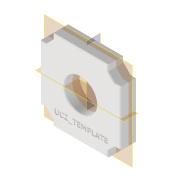
# Autodesk Inventor part: 20_Cube_Insert_Filter_25mm
Saved by Autodesk Inventor 2022 (Build 260153000, 153)
## iProperties
Created: 2019-07-01
Part Number: 20_Cube_Insert_Filter_25mm
Material: Generic
Document SubType Name: Modeling
Designer: diederichbenedict
Density: 1 g/cm^3
Appearance: Default
Author: diederichbenedict
Autodesk Inventor part; units mm, degrees
ref_plane "YZ Plane" through (0, 0, 0) normal (1, 0, 0) x (0, 1, 0)
ref_plane "XZ Plane" through (0, 0, 0) normal (0, 1, 0) x (-1, 0, 0)
ref_plane "Work Plane1" through (-56.3599, 0, 22) normal (0, 0, -1) x (-1, 0, 0)
sketch "Sketch1" plane through (-56.3599, 0, 22) normal (0, 0, -1) x (-1, 0, 0)
  line L0 (-4.0299, -0.3538) -> (-2.2322, 1.4439) construction
  arc A0 (-1.4439, 2.2322) -> (-2.2322, 1.4439) centre (-0.9299, 0.9299) ccw construction
  line L1 (-1.4439, 2.2322) -> (0.3538, 4.0299) construction
  line L2 (-37.8299, 42.8299) -> (-37.8299, 37.8299) construction
  line L3 (-37.8299, 37.8299) -> (-42.9208, 37.8299) construction
  line L4 (-37.8299, 42.2137) -> (-37.8299, 45.8299) construction
  line L5 (-37.8299, 45.8299) -> (-4.0299, 45.8299) construction
  line L6 (-4.0299, 45.8299) -> (-4.0299, 42.2137) construction
  line L7 (-4.0299, 4.0299) -> (0.3538, 4.0299) projected
  circle A1 centre (-20.9299, 20.9299) radius 17.5 projected
  line L8 (-20.9299, 58.9723) -> (17.1124, 20.9299) construction
  line L9 (17.1124, 20.9299) -> (-20.9299, -17.1124) construction
  line L10 (-20.9299, -17.1124) -> (-58.9723, 20.9299) construction
  line L11 (-58.9723, 20.9299) -> (-20.9299, 58.9723) construction
  line L12 (-20.9299, 58.9723) -> (-20.9299, -17.1124) construction
  line L13 (17.1124, 20.9299) -> (-58.9723, 20.9299) construction
  line L14 (-20.9299, 58.9723) -> (32.8701, 58.9723) construction
  line L15 (-43.4299, 43.4299) -> (1.5701, 43.4299) construction
  line L16 (1.5701, 43.4299) -> (1.5701, -1.5701) construction
  line L17 (1.5701, -1.5701) -> (-43.4299, -1.5701) construction
  line L18 (-43.4299, -1.5701) -> (-43.4299, 43.4299) construction
  line L19 (-43.4299, 43.4299) -> (1.5701, -1.5701) construction
  line L20 (1.5701, 43.4299) -> (-43.4299, -1.5701) construction
  line L21 (-43.4299, 5.3876) -> (-43.4299, 36.4723)
  line L22 (-43.4299, 36.4723) -> (-36.4723, 43.4299)
  line L23 (-36.4723, 43.4299) -> (-5.3876, 43.4299)
  line L24 (-5.3876, 43.4299) -> (1.5701, 36.4723)
  line L25 (1.5701, 36.4723) -> (1.5701, 5.3876)
  line L26 (1.5701, 5.3876) -> (-5.3876, -1.5701)
  line L27 (-5.3876, -1.5701) -> (-36.4723, -1.5701)
  line L28 (-36.4723, -1.5701) -> (-43.4299, 5.3876)
  line L29 (-4.0299, 42.2137) -> (-37.8299, 42.2137) projected
  line L30 (-4.0299, -0.3538) -> (-4.0299, 4.0299) projected
  circle A2 centre (-20.9299, 20.9299) radius 1.5
  line L31 (-10.9299, 10.9299) -> (-30.9299, 10.9299) construction
  line L32 (-30.9299, 10.9299) -> (-30.9299, 30.9299) construction
  line L33 (-30.9299, 30.9299) -> (-10.9299, 30.9299) construction
  line L34 (-10.9299, 30.9299) -> (-10.9299, 10.9299) construction
  line L35 (-10.9299, 10.9299) -> (-30.9299, 30.9299) construction
  line L36 (-30.9299, 10.9299) -> (-10.9299, 30.9299) construction
  circle A3 centre (-30.9299, 30.9299) radius 1.4
  circle A4 centre (-30.9299, 10.9299) radius 1.4
  circle A5 centre (-10.9299, 10.9299) radius 1.4
  line L37 (-45.8299, 37.8299) -> (-42.0723, 37.8299) construction
  line L38 (-42.1723, 37.7299) -> (-45.8299, 37.7299)
  line L39 (-45.8299, 37.7299) -> (-45.8299, 4.1299)
  line L40 (-45.8299, 4.1299) -> (-42.1723, 4.1299)
  line L41 (-42.1723, 4.1299) -> (-42.1723, 37.7299)
  line L42 (-45.8299, 4.0299) -> (-42.0723, 4.0299) construction
  line L43 (-45.8299, 37.8299) -> (-42.0723, 37.8299) projected
  line L44 (-37.7299, 45.8299) -> (-4.1299, 45.8299)
  line L45 (-4.1299, 45.8299) -> (-4.1299, 42.1723)
  line L46 (-4.1299, 42.1723) -> (-37.7299, 42.1723)
  line L47 (-37.7299, 42.1723) -> (-37.7299, 45.8299)
  line L48 (0.4701, 37.8299) -> (0.4701, 4.0299) construction
  line L49 (0.4701, 4.0299) -> (3.9701, 4.0299) construction
  line L50 (3.9701, 37.8299) -> (3.9701, 4.0299) construction
  line L51 (0.4701, 37.8299) -> (3.9701, 37.8299) construction
  line L52 (-45.8299, -3.9701) -> (-4.0299, -3.9701) construction
  line L53 (0.3124, 37.7299) -> (3.9701, 37.7299)
  line L54 (3.9701, 37.7299) -> (3.9701, 4.1299)
  line L55 (3.9701, 4.1299) -> (0.3124, 4.1299)
  line L56 (0.3124, 4.1299) -> (0.3124, 37.7299)
  line L57 (-4.1713, -0.3538) -> (-37.7299, -0.3538)
  line L58 (-37.7299, -0.3538) -> (-37.7299, -3.9701)
  line L59 (-37.7299, -3.9701) -> (-4.1713, -3.9701)
  line L60 (-4.1713, -3.9701) -> (-4.1713, -0.3538)
  point P0 (-37.8299, 4.0299)
  dimension "d18" = 53.8
  dimension "d19" = 45
  dimension "d20" = 53.8
  dimension "d21" = 45
  dimension "d22" = 45
  dimension "d30" = 20
  dimension "d31" = 20
  dimension "d32" = 2.8
  dimension "d33" = 2.8
  dimension "d34" = 2.8
  dimension "d35" = 3
  dimension "d36" = 0.1
  dimension "d37" = 0.1
  dimension "d38" = 0.1
  dimension "d39" = 0.1
  constraints: 86 end point, 21 point on line, 14 parallel, 8 perpendicular, 7 horizontal, 7 midpoint, 4 centre point, 4 coincident, 1 equal length
  measures "d18" distance of L8.start L8.end
  measures "d19" angle of L8 L14
  measures "d20" distance of L8.end L9.end
  measures "d21" distance of L16.end L17.end
  measures "d22" distance of L15.end L16.end
  measures "d30" distance of L32.end L33.end
  measures "d31" distance of L31.end L32.end
  measures "d32" diameter of A3
  measures "d33" diameter of A4
  measures "d34" diameter of A5
  measures "d35" diameter of A2
  measures "d36" distance between parallel lines of L38 L43
  measures "d37" distance between parallel lines of L40 L42
  measures "d38" distance between parallel lines of L45 L6
  measures "d39" distance between parallel lines of L4 L47
extrude "Extrusion1" add sketch "Sketch1" along normal blind 10 contours L30 L26 L57 L28 L41 L22 L46 L24 L56 L7 | L7 L26 L30 | L56 L24 L25 L26 | L26 L25 L24 L53 L54 L55 | L60 L59 L58 L57 L28 L27 L26 | L26 L27 L28 L57 | L46 L22 L29 L24 | L24 L29 L45 | L40 L39 L38 L22 L21 L28 | L28 L21 L22 L41 | L29 L22 L23 L24 | L24 L23 L22 L29 L47 L44 L45 | L47 L29 L22 | A1 | A2 | A3 | A4 | A5
sketch "Skizze4" plane through (-56.3599, 0, 12) normal (0, 0, -1) x (-1, 0, 0)
  line L0 (-37.7299, 42.1723) -> (-42.1723, 37.7299) projected
  line L1 (-42.1723, 37.7299) -> (-45.8299, 37.7299) projected
  line L2 (-45.8299, 37.7299) -> (-45.8299, 4.1299) construction
  line L3 (-45.8299, 4.1299) -> (-42.1723, 4.1299) projected
  line L4 (-42.1723, 4.1299) -> (-37.6885, -0.3538) projected
  line L5 (-37.6885, -0.3538) -> (-37.7299, -0.3538) projected
  line L6 (-37.7299, -0.3538) -> (-37.7299, -3.9701) projected
  line L7 (-37.7299, -3.9701) -> (-4.1713, -3.9701) construction
  line L8 (-4.1713, -3.9701) -> (-4.1713, -0.3538) projected
  line L9 (-4.1713, -0.3538) -> (0.3124, 4.1299) projected
  line L10 (0.3124, 4.1299) -> (3.9701, 4.1299) projected
  line L11 (3.9701, 4.1299) -> (3.9701, 37.7299) construction
  line L12 (3.9701, 37.7299) -> (0.3124, 37.7299) projected
  line L13 (0.3124, 37.7299) -> (-4.1299, 42.1723) projected
  line L14 (-4.1299, 42.1723) -> (-4.1299, 45.8299) projected
  line L15 (-4.1299, 45.8299) -> (-37.7299, 45.8299) construction
  line L16 (-37.7299, 45.8299) -> (-37.7299, 42.1723) projected
  line L17 (-37.9299, 46.0299) -> (-3.9299, 46.0299) construction
  line L18 (-3.9299, 46.0299) -> (-3.9299, 42.2551)
  line L19 (-3.9299, 42.2551) -> (0.3953, 37.9299)
  line L20 (0.3953, 37.9299) -> (4.1701, 37.9299)
  line L21 (4.1701, 37.9299) -> (4.1701, 3.9299) construction
  line L22 (4.1701, 3.9299) -> (0.3953, 3.9299)
  line L23 (0.3953, 3.9299) -> (-3.9713, -0.4367)
  line L24 (-3.9713, -0.4367) -> (-3.9713, -4.1701)
  line L25 (-3.9713, -4.1701) -> (-37.9299, -4.1701) construction
  line L26 (-37.9299, -4.1701) -> (-37.9299, -0.3953)
  line L27 (-37.9299, -0.3953) -> (-42.2551, 3.9299)
  line L28 (-42.2551, 3.9299) -> (-46.0299, 3.9299)
  line L29 (-46.0299, 3.9299) -> (-46.0299, 37.9299) construction
  line L30 (-46.0299, 37.9299) -> (-42.2551, 37.9299)
  line L31 (-42.2551, 37.9299) -> (-37.9299, 42.2551)
  line L32 (-37.9299, 42.2551) -> (-37.9299, 46.0299)
  line L33 (-45.8299, 37.7299) -> (-45.8299, 37.9299)
  line L34 (-4.1299, 45.8299) -> (-37.7299, 45.8299) projected
  line L35 (-37.7299, 45.8299) -> (-37.9299, 45.8299)
  line L36 (-4.1299, 45.8299) -> (-3.9299, 45.8299)
  line L37 (3.9701, 37.7299) -> (3.9701, 37.9299)
  line L38 (3.9701, 4.1299) -> (3.9701, 37.7299) projected
  line L39 (3.9701, 4.1299) -> (3.9701, 3.9299)
  line L40 (-4.1713, -3.9701) -> (-3.9713, -3.9701)
  line L41 (-37.7299, -3.9701) -> (-37.9299, -3.9701)
  line L42 (-45.8299, 4.1299) -> (-45.8299, 3.9299)
  point P0 (-56.3599, 0)
  dimension "d40" = 0.2
  constraints: 48 end point, 12 point on line, 4 perpendicular, 15 other
  measures "d40" distance between parallel lines of L15 L17
extrude "IM_offset" add sketch "Skizze4" against normal up to surface (10 mm away)
ref_plane "Arbeitsebene5" through (-35.4299, 3.9299, 22) normal (-1, 0, 0) x (0, 0, 1)
ref_plane "Arbeitsebene6" through (-18.4299, 20.9299, 22) normal (0, 1, 0) x (-1, 0, 0)
sketch "Skizze31" plane through (-56.3599, 0, 12) normal (0, 0, -1) x (-1, 0, 0)
  line L0 (3.9701, 3.9299) -> (3.9701, 37.9299) projected
  line L1 (3.9701, 37.9299) -> (0.3953, 37.9299) projected
  line L2 (0.3953, 37.9299) -> (-3.9299, 42.2551) projected
  line L3 (-3.9299, 42.2551) -> (-3.9299, 45.8299) projected
  line L4 (-3.9299, 45.8299) -> (-37.9299, 45.8299) projected
  line L5 (-37.9299, 45.8299) -> (-37.9299, 42.2551) projected
  line L6 (-37.9299, 42.2551) -> (-42.2551, 37.9299) projected
  line L7 (-42.2551, 37.9299) -> (-45.8299, 37.9299) projected
  line L8 (-45.8299, 37.9299) -> (-45.8299, 3.9299) projected
  line L9 (-42.2551, 3.9299) -> (-45.8299, 3.9299) projected
  line L10 (-37.9299, -0.3953) -> (-42.2551, 3.9299) projected
  line L11 (-37.9299, -3.9701) -> (-37.9299, -0.3953) projected
  line L12 (-3.9713, -3.9701) -> (-37.9299, -3.9701) projected
  line L13 (-3.9713, -3.9701) -> (-3.9713, -0.4367) projected
  line L14 (-3.9713, -0.4367) -> (0.3953, 3.9299) projected
  line L15 (0.3953, 3.9299) -> (3.9701, 3.9299) projected
  circle A0 centre (-20.9506, 20.9092) radius 10
  point P0 (-56.3599, 0)
  dimension "d181" = 20
  constraints: 1 centre point
  measures "d181" diameter of A0
extrude "Extrusion26" cut sketch "Skizze31" against normal blind 10 contours A0
chamfer "Fase2" distance 0.5 angle 45 34 edges at (-35.4299, 45.8299, 22) (-18.4299, 44.0425, 22) (-16.2673, 40.0925, 22) (-12.3173, 37.9299, 22) (-10.5299, 20.9299, 22) (-12.3173, 3.9299, 22) (-16.2673, 1.7673, 22) (-18.4299, -2.1827, 22) (-35.4092, -3.9701, 22) (-52.3885, -2.2034, 22) (-54.5718, 1.7466, 22) (-58.5425, 3.9299, 22) (-60.3299, 20.9299, 22) (-58.5425, 37.9299, 22) (-54.5925, 40.0925, 22) (-54.5718, 1.7466, 12) (-58.5425, 3.9299, 12) (-60.3299, 20.9299, 12) (-52.3885, -2.2034, 12) (-35.4092, -3.9701, 12) (-18.4299, -2.1827, 12) (-16.2673, 1.7673, 12) (-12.3173, 3.9299, 12) (-10.5299, 20.9299, 12) (-12.3173, 37.9299, 12) (-16.2673, 40.0925, 12) (-18.4299, 44.0425, 12) (-35.4299, 45.8299, 12) (-52.4299, 44.0425, 12) (-54.5925, 40.0925, 12) (-58.5425, 37.9299, 12) (-25.4092, 20.9092, 12) (-25.4092, 20.9092, 22) (-52.4299, 44.0425, 22)
sketch "Skizze32" plane through (-56.3599, 0, 22) normal (0, 0, 1) x (1, 0, 0)
  line L0 (4.8056, 6.489) -> (64.0062, 6.489) construction
  line L1 (64.0062, 6.489) -> (64.0062, -0.9654) construction
  line L2 (64.0062, -0.9654) -> (4.8056, -0.9654) construction
  line L3 (4.8056, -0.9654) -> (4.8056, 6.489) construction
  spline S0 degree 2 poles (6.3553, 3.3155) (5.7398, 3.3155) (5.0774, 3.9087) (5.0774, 4.4821) knots 0 0 0 1 2 2 2
  line L4 (5.0774, 4.4821) -> (5.0774, 6.4297)
  line L5 (5.0774, 6.4297) -> (5.8436, 6.4297)
  line L6 (5.8436, 6.4297) -> (5.8436, 4.5266)
  spline S1 degree 2 poles (5.8436, 4.5266) (5.8436, 4.2077) (6.0834, 3.8963) (6.3553, 3.8963) knots 0 0 0 1 2 2 2
  spline S2 degree 2 poles (6.3553, 3.8963) (6.6197, 3.8963) (6.8669, 4.1954) (6.8669, 4.5266) knots 0 0 0 1 2 2 2
  line L7 (6.8669, 4.5266) -> (6.8669, 6.4297)
  line L8 (6.8669, 6.4297) -> (7.6331, 6.4297)
  line L9 (7.6331, 6.4297) -> (7.6331, 4.4845)
  spline S3 degree 2 poles (7.6331, 4.4845) (7.6331, 3.921) (6.988, 3.3155) (6.3553, 3.3155) knots 0 0 0 1 2 2 2
  spline S4 degree 2 poles (9.5363, 3.3204) (8.8492, 3.3204) (8.0434, 4.1509) (8.0434, 4.9022) knots 0 0 0 1 2 2 2
  spline S5 degree 2 poles (8.0434, 4.9022) (8.0434, 5.6264) (8.8516, 6.489) (9.5387, 6.489) knots 0 0 0 1 2 2 2
  spline S6 degree 2 poles (9.5387, 6.489) (9.7192, 6.489) (10.0108, 6.447) (10.1443, 6.4124) knots 0 0 0 1 2 2 2
  spline S7 degree 2 poles (10.1443, 6.4124) (10.2481, 6.3803) (10.4928, 6.274) (10.5694, 6.2345) knots 0 0 0 1 2 2 2
  line L10 (10.5694, 6.2345) -> (10.5694, 5.5078)
  line L11 (10.5694, 5.5078) -> (10.4928, 5.5078)
  spline S8 degree 2 poles (10.4928, 5.5078) (10.4359, 5.5572) (10.2679, 5.6956) (10.1616, 5.7599) knots 0 0 0 1 2 2 2
  spline S9 degree 2 poles (10.1616, 5.7599) (10.0553, 5.8266) (9.8007, 5.9181) (9.6599, 5.9181) knots 0 0 0 1 2 2 2
  spline S10 degree 2 poles (9.6599, 5.9181) (9.4943, 5.9181) (9.2199, 5.8143) (9.0939, 5.6833) knots 0 0 0 1 2 2 2
  spline S11 degree 2 poles (9.0939, 5.6833) (8.9802, 5.5671) (8.8343, 5.1692) (8.8343, 4.8998) knots 0 0 0 1 2 2 2
  spline S12 degree 2 poles (8.8343, 4.8998) (8.8343, 4.6155) (8.9851, 4.2275) (9.1087, 4.1089) knots 0 0 0 1 2 2 2
  spline S13 degree 2 poles (9.1087, 4.1089) (9.2273, 3.9927) (9.519, 3.8913) (9.6648, 3.8913) knots 0 0 0 1 2 2 2
  spline S14 degree 2 poles (9.6648, 3.8913) (9.8156, 3.8913) (10.0899, 3.9927) (10.1838, 4.0545) knots 0 0 0 1 2 2 2
  spline S15 degree 2 poles (10.1838, 4.0545) (10.2877, 4.1163) (10.4434, 4.2473) (10.5002, 4.2992) knots 0 0 0 1 2 2 2
  line L12 (10.5002, 4.2992) -> (10.5694, 4.2992)
  line L13 (10.5694, 4.2992) -> (10.5694, 3.5824)
  spline S16 degree 2 poles (10.5694, 3.5824) (10.4854, 3.5428) (10.2654, 3.444) (10.1468, 3.4094) knots 0 0 0 1 2 2 2
  spline S17 degree 2 poles (10.1468, 3.4094) (10.0034, 3.3649) (9.7538, 3.3204) (9.5363, 3.3204) knots 0 0 0 1 2 2 2
  line L14 (13.2561, 3.3797) -> (11.0143, 3.3797)
  line L15 (11.0143, 3.3797) -> (11.0143, 3.8765)
  spline S18 degree 2 poles (11.0143, 3.8765) (11.2986, 4.1039) (11.7533, 4.5043) (11.9239, 4.6847) knots 0 0 0 1 2 2 2
  spline S19 degree 2 poles (11.9239, 4.6847) (12.1488, 4.9195) (12.349, 5.2779) (12.349, 5.4658) knots 0 0 0 1 2 2 2
  spline S20 degree 2 poles (12.349, 5.4658) (12.349, 5.6783) (12.0944, 5.9057) (11.867, 5.9057) knots 0 0 0 1 2 2 2
  spline S21 degree 2 poles (11.867, 5.9057) (11.7509, 5.9057) (11.5432, 5.8489) (11.437, 5.8044) knots 0 0 0 1 2 2 2
  spline S22 degree 2 poles (11.437, 5.8044) (11.3332, 5.7574) (11.1849, 5.6586) (11.1478, 5.6339) knots 0 0 0 1 2 2 2
  line L16 (11.1478, 5.6339) -> (11.0885, 5.6339)
  line L17 (11.0885, 5.6339) -> (11.0885, 6.2987)
  spline S23 degree 2 poles (11.0885, 6.2987) (11.217, 6.3605) (11.7657, 6.489) (12.0203, 6.489) knots 0 0 0 1 2 2 2
  spline S24 degree 2 poles (12.0203, 6.489) (12.564, 6.489) (13.1226, 6.0046) (13.1226, 5.5671) knots 0 0 0 1 2 2 2
  spline S25 degree 2 poles (13.1226, 5.5671) (13.1226, 5.2977) (12.868, 4.7787) (12.5739, 4.4821) knots 0 0 0 1 2 2 2
  spline S26 degree 2 poles (12.5739, 4.4821) (12.3885, 4.2992) (12.04, 4.0149) (11.9634, 3.9556) knots 0 0 0 1 2 2 2
  line L18 (11.9634, 3.9556) -> (13.2561, 3.9556)
  line L19 (13.2561, 3.9556) -> (13.2561, 3.3797)
  line L20 (16.0812, 2.6728) -> (13.3451, 2.6728)
  line L21 (13.3451, 2.6728) -> (13.3451, 3.0856)
  line L22 (13.3451, 3.0856) -> (16.0812, 3.0856)
  line L23 (16.0812, 3.0856) -> (16.0812, 2.6728)
  line L24 (16.9512, 3.3797) -> (16.9512, 5.8489)
  line L25 (16.9512, 5.8489) -> (16.049, 5.8489)
  line L26 (16.049, 5.8489) -> (16.049, 6.4297)
  line L27 (16.049, 6.4297) -> (18.6195, 6.4297)
  line L28 (18.6195, 6.4297) -> (18.6195, 5.8489)
  line L29 (18.6195, 5.8489) -> (17.7174, 5.8489)
  line L30 (17.7174, 5.8489) -> (17.7174, 3.3797)
  line L31 (17.7174, 3.3797) -> (16.9512, 3.3797)
  line L32 (18.9334, 3.3797) -> (18.9334, 6.4297)
  line L33 (18.9334, 6.4297) -> (20.9948, 6.4297)
  line L34 (20.9948, 6.4297) -> (20.9948, 5.8489)
  line L35 (20.9948, 5.8489) -> (19.6947, 5.8489)
  line L36 (19.6947, 5.8489) -> (19.6947, 5.3125)
  line L37 (19.6947, 5.3125) -> (20.8934, 5.3125)
  line L38 (20.8934, 5.3125) -> (20.8934, 4.7317)
  line L39 (20.8934, 4.7317) -> (19.6947, 4.7317)
  line L40 (19.6947, 4.7317) -> (19.6947, 3.9606)
  line L41 (19.6947, 3.9606) -> (20.9948, 3.9606)
  line L42 (20.9948, 3.9606) -> (20.9948, 3.3797)
  line L43 (20.9948, 3.3797) -> (18.9334, 3.3797)
  line L44 (24.6281, 3.3797) -> (23.8668, 3.3797)
  line L45 (23.8668, 3.3797) -> (23.8668, 5.4015)
  line L46 (23.8668, 5.4015) -> (23.3132, 4.0965)
  line L47 (23.3132, 4.0965) -> (22.7892, 4.0965)
  line L48 (22.7892, 4.0965) -> (22.2355, 5.4015)
  line L49 (22.2355, 5.4015) -> (22.2355, 3.3797)
  line L50 (22.2355, 3.3797) -> (21.5138, 3.3797)
  line L51 (21.5138, 3.3797) -> (21.5138, 6.4297)
  line L52 (21.5138, 6.4297) -> (22.3962, 6.4297)
  line L53 (22.3962, 6.4297) -> (23.0734, 4.9245)
  line L54 (23.0734, 4.9245) -> (23.7457, 6.4297)
  line L55 (23.7457, 6.4297) -> (24.6281, 6.4297)
  line L56 (24.6281, 6.4297) -> (24.6281, 3.3797)
  spline S27 degree 2 poles (27.6064, 5.4683) (27.6064, 5.2557) (27.4705, 4.8701) (27.3444, 4.7416) knots 0 0 0 1 2 2 2
  spline S28 degree 2 poles (27.3444, 4.7416) (27.2678, 4.66) (27.08, 4.5266) (26.9687, 4.4796) knots 0 0 0 1 2 2 2
  spline S29 degree 2 poles (26.9687, 4.4796) (26.855, 4.4326) (26.5906, 4.3783) (26.4274, 4.3783) knots 0 0 0 1 2 2 2
  line L57 (26.4274, 4.3783) -> (26.027, 4.3783)
  line L58 (26.027, 4.3783) -> (26.027, 3.3797)
  line L59 (26.027, 3.3797) -> (25.2608, 3.3797)
  line L60 (25.2608, 3.3797) -> (25.2608, 6.4297)
  line L61 (25.2608, 6.4297) -> (26.4447, 6.4297)
  spline S30 degree 2 poles (26.4447, 6.4297) (26.7067, 6.4297) (27.0898, 6.3333) (27.2456, 6.2295) knots 0 0 0 1 2 2 2
  spline S31 degree 2 poles (27.2456, 6.2295) (27.4186, 6.1134) (27.6064, 5.7327) (27.6064, 5.4683) knots 0 0 0 1 2 2 2
  spline S32 degree 2 poles (26.8204, 5.4485) (26.8204, 5.5795) (26.6968, 5.7648) (26.6128, 5.7995) knots 0 0 0 1 2 2 2
  spline S33 degree 2 poles (26.6128, 5.7995) (26.5041, 5.8464) (26.3063, 5.8612) (26.1358, 5.8612) knots 0 0 0 1 2 2 2
  line L62 (26.1358, 5.8612) -> (26.027, 5.8612)
  line L63 (26.027, 5.8612) -> (26.027, 4.9467)
  line L64 (26.027, 4.9467) -> (26.0814, 4.9467)
  spline S34 degree 2 poles (26.0814, 4.9467) (26.1877, 4.9467) (26.3805, 4.9517) (26.4522, 4.964) knots 0 0 0 1 2 2 2
  spline S35 degree 2 poles (26.4522, 4.964) (26.5139, 4.9739) (26.6499, 5.0332) (26.687, 5.0703) knots 0 0 0 1 2 2 2
  spline S36 degree 2 poles (26.687, 5.0703) (26.7661, 5.1445) (26.8204, 5.3101) (26.8204, 5.4485) knots 0 0 0 1 2 2 2
  line L65 (30.0509, 3.3797) -> (28.0167, 3.3797)
  line L66 (28.0167, 3.3797) -> (28.0167, 6.4297)
  line L67 (28.0167, 6.4297) -> (28.7829, 6.4297)
  line L68 (28.7829, 6.4297) -> (28.7829, 3.9606)
  line L69 (28.7829, 3.9606) -> (30.0509, 3.9606)
  line L70 (30.0509, 3.9606) -> (30.0509, 3.3797)
  line L71 (30.0879, 3.3797) -> (31.1186, 6.4297)
  line L72 (31.1186, 6.4297) -> (31.954, 6.4297)
  line L73 (31.954, 6.4297) -> (32.9847, 3.3797)
  line L74 (32.9847, 3.3797) -> (32.1962, 3.3797)
  line L75 (32.1962, 3.3797) -> (32.0059, 4.0026)
  line L76 (32.0059, 4.0026) -> (31.0469, 4.0026)
  line L77 (31.0469, 4.0026) -> (30.8541, 3.3797)
  line L78 (30.8541, 3.3797) -> (30.0879, 3.3797)
  line L79 (31.8379, 4.5562) -> (31.5264, 5.5646)
  line L80 (31.5264, 5.5646) -> (31.2125, 4.5562)
  line L81 (31.2125, 4.5562) -> (31.8379, 4.5562)
  line L82 (33.8745, 3.3797) -> (33.8745, 5.8489)
  line L83 (33.8745, 5.8489) -> (32.9723, 5.8489)
  line L84 (32.9723, 5.8489) -> (32.9723, 6.4297)
  line L85 (32.9723, 6.4297) -> (35.5428, 6.4297)
  line L86 (35.5428, 6.4297) -> (35.5428, 5.8489)
  line L87 (35.5428, 5.8489) -> (34.6407, 5.8489)
  line L88 (34.6407, 5.8489) -> (34.6407, 3.3797)
  line L89 (34.6407, 3.3797) -> (33.8745, 3.3797)
  line L90 (35.8567, 3.3797) -> (35.8567, 6.4297)
  line L91 (35.8567, 6.4297) -> (37.9181, 6.4297)
  line L92 (37.9181, 6.4297) -> (37.9181, 5.8489)
  line L93 (37.9181, 5.8489) -> (36.618, 5.8489)
  line L94 (36.618, 5.8489) -> (36.618, 5.3125)
  line L95 (36.618, 5.3125) -> (37.8167, 5.3125)
  line L96 (37.8167, 5.3125) -> (37.8167, 4.7317)
  line L97 (37.8167, 4.7317) -> (36.618, 4.7317)
  line L98 (36.618, 4.7317) -> (36.618, 3.9606)
  line L99 (36.618, 3.9606) -> (37.9181, 3.9606)
  line L100 (37.9181, 3.9606) -> (37.9181, 3.3797)
  line L101 (37.9181, 3.3797) -> (35.8567, 3.3797)
  point P0 (56.3599, 0)
  constraints: 2 other
extrude "Extrusion27" cut sketch "Skizze32" against normal blind 1
ref_plane "Arbeitsebene9" through (-56.3599, 0, 17) normal (0, 0, 1) x (1, 0, 0)
body "Solid1"
